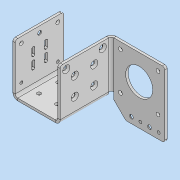
# Autodesk Inventor part: Gantry_Angle
Saved by Autodesk Inventor 2020 (Build 240168000, 168)
## iProperties
Created: 2021-05-02
Part Number: Gantry_Angle
Material: 一般
Document SubType Name: Sheet Metal
Designer: ken113
Density: 1 g/cm^3
Sheet Metal Rule: Default_mm
Appearance: 既定
Author: ken113
Autodesk Inventor part; units mm, degrees
ref_plane "YZ Plane" through (0, 0, 0) normal (1, 0, 0) x (0, 1, 0)
ref_plane "XZ Plane" through (0, 0, 0) normal (0, 1, 0) x (-1, 0, 0)
ref_plane "XY Plane" through (0, 0, 0) normal (0, 0, 1) x (1, 0, 0)
sketch "スケッチ1" plane through (0, 0, 0) normal (0, 1, 0) x (-1, 0, 0)
  line L0 (15, 20) -> (-20, 20)
  line L1 (-20, 20) -> (-20, -20)
  line L2 (-20, -20) -> (15, -20)
  line L3 (15, -20) -> (15, 20)
  point P0 (0, 0)
  dimension "d0" = 15
  dimension "d1" = 40
  dimension "d2" = 20
  dimension "d3" = 20
  measures "d0" distance from line of L3 point (0, 0)
  measures "d1" distance of L0.end L1.end
  measures "d2" distance from line of point (0, 0) L1
  measures "d3" distance from line of point (0, 0) L2
extrude "プレート1" add sketch "スケッチ1" along normal blind 2
sketch "スケッチ2" plane through (0, 2, 0) normal (0, 1, 0) x (1, 0, 0)
  line L0 (7.5, 8) -> (-7.5, 8)
  line L1 (-7.5, 8) -> (-7.5, -8)
  line L2 (-7.5, -8) -> (7.5, -8)
  line L3 (7.5, -8) -> (7.5, 8)
  line L4 (7.5, 8) -> (-7.5, -8) construction
  line L5 (-7.5, 8) -> (7.5, -8) construction
  point P0 (0, 0)
  dimension "d5" = 15
  dimension "d6" = 16
  constraints: 12 end point, 2 midpoint, 2 parallel, 1 horizontal, 1 perpendicular
  measures "d5" distance of L2.end L1.end
  measures "d6" distance of L1.end L0.end
hole "穴1" at (-7.5, 2, 8) at (7.5, 2, 8) at (7.5, 2, -8) at (-7.5, 2, -8) direction (0, -1, 0) diameter 3.2 depth 2 tip angle 118
sketch "スケッチ3" plane through (-15, 2, 20) normal (-1, 0, 0) x (0, -1, 0)
  line L0 (0, -40) -> (0, 0)
  line L1 (0, 0) -> (-40.5, 0)
  line L2 (-40.5, 0) -> (-40.5, -40)
  line L3 (-40.5, -40) -> (0, -40)
  constraints: 6 end point, 1 horizontal, 1 perpendicular, 1 vertical
edge flange "フランジ1" height 42.5 angle 90 thickness 2 bend radius 2 thickness toward (-1, 0, 0) relief straight relief width 2 relief depth 1 corner gap 2 corner form 0 edges at (-15, 2, 0) (20, 2, 0) wall of the first edge with corners at (-15, 2, -20) (-15, 2, 20) (-15, 42.5, 20) (-15, 42.5, -20)
bend "曲げ1"
corner "コーナー1"
sketch "スケッチ5" plane through (22, 42.5, 20) normal (1, 0, 0) x (0, 0, -1)
  line L0 (12, -28) -> (28, -28)
  line L1 (28, -28) -> (28, -13)
  line L2 (28, -13) -> (12, -13)
  line L3 (12, -13) -> (12, -28)
  line L4 (12, -28) -> (28, -13) construction
  line L5 (28, -28) -> (12, -13) construction
  line L6 (0, -38.5) -> (40, -38.5) projected
  point P0 (20, -42.5)
  point P1 (20, -20.5)
  point P2 (20, -20.5)
  dimension "d34" = 16
  dimension "d35" = 15
  dimension "d36" = 10.5
  constraints: 12 end point, 3 midpoint, 2 parallel, 1 horizontal, 1 perpendicular, 1 vertical alignment
  measures "d34" distance of L1.end L2.end
  measures "d35" distance of L0.end L1.end
  measures "d36" distance between parallel lines of L0 L6
hole "穴2" at (22, 29.5, 8) at (22, 29.5, -8) at (22, 14.5, -8) at (22, 14.5, 8) direction (-1, 0, 0) diameter 3.2 depth 2 tip angle 118 countersink diameter 6 countersink angle 90
sketch "スケッチ6" plane through (24, 42.5, -22) normal (0, 0, -1) x (-1, 0, 0)
  line L0 (0, -38.5) -> (0, 0)
  line L1 (0, 0) -> (-42, 0)
  line L2 (-42, 0) -> (-42, -38.5)
  line L3 (-42, -38.5) -> (0, -38.5)
  constraints: 6 end point, 1 horizontal, 1 perpendicular, 1 vertical
edge flange "フランジ3" height 46 angle 90 thickness 2 bend radius 2 thickness toward (0, 0, -1) relief straight relief width 2 relief depth 1 edges at (22, 23.25, -20) wall of the first edge with corners at (24, 4, -22) (24, 42.5, -22) (66, 42.5, -22) (66, 4, -22)
bend "曲げ3"
corner "コーナー3"
sketch "スケッチ7" plane through (66, 4, -24) normal (0, -1, 0) x (1, 0, 0)
  line L0 (-42, 2) -> (-42, 0) projected
  line L1 (-42, 0) -> (0, 0) projected
  line L2 (0, 2) -> (0, 0) projected
  line L3 (0, 2) -> (-42, 2) projected
  point P0 (-66, 24)
extrude "押し出し1" add sketch "スケッチ7" along normal blind 15.5
sketch "スケッチ8" plane through (66, 42.5, -24) normal (0, 0, -1) x (-1, 0, 0)
  circle A0 centre (21, -21) radius 11.15
  line L0 (42, -38.5) -> (42, 0) projected
  line L1 (5.5, -36.5) -> (36.5, -36.5)
  line L2 (36.5, -36.5) -> (36.5, -5.5)
  line L3 (36.5, -5.5) -> (5.5, -5.5)
  line L4 (5.5, -5.5) -> (5.5, -36.5)
  line L5 (5.5, -36.5) -> (36.5, -5.5) construction
  line L6 (36.5, -36.5) -> (5.5, -5.5) construction
  circle A1 centre (5.5, -5.5) radius 1.6
  circle A2 centre (36.5, -5.5) radius 1.6
  circle A3 centre (36.5, -36.5) radius 1.6
  circle A4 centre (5.5, -36.5) radius 1.6
  line L7 (0, 0) -> (42, 0) projected
  point P0 (66, -42.5)
  dimension "d56" = 22.3
  dimension "d57" = 21
  dimension "d58" = 31
  dimension "d59" = 31
  dimension "d60" = 3.2
  dimension "d61" = 3.2
  dimension "d62" = 3.2
  dimension "d63" = 3.2
  dimension "d66" = 21
  constraints: 12 end point, 5 centre point, 4 coincident, 2 midpoint, 2 parallel, 1 horizontal, 1 perpendicular
  measures "d56" diameter of A0
  measures "d57" distance from line of A0.centre L0
  measures "d58" distance of L3.end L2.end
  measures "d59" distance of L2.end L1.end
  measures "d60" diameter of A1
  measures "d61" diameter of A2
  measures "d62" diameter of A3
  measures "d63" diameter of A4
  measures "d66" distance from line of L7 A0.centre
extrude "押し出し2" cut sketch "スケッチ8" against normal blind 25.5 contours A0 | L4 A4 L1 | L1 A4 L4 | A3 L2 L1 | L1 L2 A3 | A1 L3 L4 | L4 L3 A1 | A2 L3 L2 | L2 L3 A2
sketch "スケッチ9" plane through (66, 42.5, -24) normal (0, 0, -1) x (-1, 0, 0)
  circle A0 centre (5.5, -36.5) radius 1.6 projected
  circle A1 centre (36.5, -36.5) radius 1.6 projected
  circle A2 centre (5.5, -5.5) radius 1.6 projected
  circle A3 centre (36.5, -5.5) radius 1.6 projected
  circle A4 centre (21, -21) radius 11.15 projected
  line L0 (42, -38.5) -> (42, 0) projected
  line L1 (0, 0) -> (42, 0) projected
  line L2 (0, 0) -> (0, -54) projected
  line L3 (42, -54) -> (0, -54) projected
  line L4 (42, -38.5) -> (42, -54) projected
  point P0 (66, -42.5)
  point P1 (5, -49)
  point P2 (20, -49)
  dimension "d67" = 5
  dimension "d69" = 5
  dimension "d77" = 15
  constraints: 1 horizontal alignment
  measures "d67" distance from line of point (20, -49) L3
  measures "d69" distance from line of point (5, -49) L2
  measures "d77" distance of point (20, -49) point (5, -49)
hole "穴3" at (61, -6.5, -24) at (46, -6.5, -24) direction (0, 0, 1) diameter 2.459 end through all thread size "M3x0.5" class "6H" standard "ISO Metric profile"
chamfer "面取り1" distance 10 angle 45 1 edges at (24, -11.5, -23)
sketch "スケッチ10" plane through (22, 4, 20) normal (1, 0, 0) x (0, 0, -1)
  circle A0 centre (28, 10.5) radius 3 projected
  circle A1 centre (12, 25.5) radius 3 projected
  circle A2 centre (28, 25.5) radius 3 projected
  circle A3 centre (12, 10.5) radius 3 projected
  line L0 (0, 0) -> (40, 0) projected
  line L1 (40, 38.5) -> (40, 0) projected
  line L2 (0, 38.5) -> (40, 38.5) projected
  line L3 (0, 0) -> (0, 38.5) projected
  point P0 (20, -4)
  point P1 (5, 33.5)
  point P2 (35, 33.5)
  dimension "d81" = 5
  dimension "d82" = 30
  dimension "d83" = 5
  constraints: 1 horizontal alignment
  measures "d81" distance from line of L2 point (5, 33.5)
  measures "d82" distance of point (35, 33.5) point (5, 33.5)
  measures "d83" distance from line of point (5, 33.5) L3
hole "穴4" at (22, 37.5, 15) at (22, 37.5, -15) direction (-1, 0, 0) diameter 3.2 end through all countersink diameter 6 countersink angle 90
fillet "フィレット1" radius 2 7 edges at (-16, 42.5, -20) (-16, 42.5, 20) (21, 42.5, 20) (66, 42.5, -23) (66, -11.5, -23) (34, -11.5, -23) (24, -1.5, -23)
sketch "スケッチ13" plane through (-17, 4, -20) normal (-1, 0, 0) x (0, 0, 1)
  line L0 (13.5, 26) -> (16, 26)
  line L1 (16, 26) -> (16, 19.5)
  line L2 (16, 19.5) -> (13.5, 19.5)
  line L3 (13.5, 19.5) -> (13.5, 26)
  line L4 (13.5, 16.5) -> (16, 16.5)
  line L5 (16, 16.5) -> (16, 10)
  line L6 (16, 10) -> (13.5, 10)
  line L7 (13.5, 10) -> (13.5, 16.5)
  line L8 (24, 19.5) -> (26.5, 19.5)
  line L9 (26.5, 19.5) -> (26.5, 26)
  line L10 (26.5, 26) -> (24, 26)
  line L11 (24, 26) -> (24, 19.5)
  line L12 (24, 16.5) -> (26.5, 16.5)
  line L13 (26.5, 16.5) -> (26.5, 10)
  line L14 (26.5, 10) -> (24, 10)
  line L15 (24, 10) -> (24, 16.5)
  line L16 (40, -4) -> (0, -4) projected
  line L17 (2, 38.5) -> (38, 38.5) projected
  line L18 (13.5, 26) -> (26.5, 26)
  line L19 (26.5, 26) -> (26.5, 26.25)
  line L20 (26.5, 26.25) -> (13.5, 26.25)
  line L21 (13.5, 26.25) -> (13.5, 26)
  line L22 (13.5, 16.5) -> (26.5, 16.5)
  line L23 (26.5, 16.5) -> (26.5, 16.75)
  line L24 (26.5, 16.75) -> (13.5, 16.75)
  line L25 (13.5, 16.75) -> (13.5, 16.5)
  line L26 (13.5, 19.5) -> (26.5, 19.5)
  line L27 (26.5, 19.5) -> (26.5, 19.25)
  line L28 (26.5, 19.25) -> (13.5, 19.25)
  line L29 (13.5, 19.25) -> (13.5, 19.5)
  line L30 (13.5, 10) -> (26.5, 10)
  line L31 (26.5, 10) -> (26.5, 9.75)
  line L32 (26.5, 9.75) -> (13.5, 9.75)
  line L33 (13.5, 9.75) -> (13.5, 10)
  line L34 (16, 26.25) -> (24, 26.25)
  line L35 (24, 26.25) -> (24, 9.75)
  line L36 (24, 9.75) -> (16, 9.75)
  line L37 (16, 9.75) -> (16, 26.25)
  point P0 (20, -4)
  point P1 (26.5, 26.125)
  point P2 (24, 16.75)
  point P3 (24, 19.25)
  point P4 (16, 19.25)
  point P5 (16, 9.75)
  point P6 (16, 10)
  point P7 (16, 16.5)
  point P8 (16, 16.75)
  dimension "d110" = 6.5
  dimension "d111" = 6.5
  dimension "d112" = 2.5
  dimension "d113" = 2.5
  dimension "d114" = 14
  dimension "d115" = 12.5
  dimension "d116" = 8
  dimension "d117" = 4
  dimension "d118" = 7
  dimension "d119" = 0.25
  dimension "d120" = 7
  dimension "d121" = 0.25
  constraints: 72 end point, 18 parallel, 9 horizontal, 9 perpendicular, 9 vertical alignment, 7 point on line, 4 horizontal alignment, 1 coincident, 1 midpoint
  measures "d110" distance of L8.end L9.end
  measures "d111" distance of L12.end L13.end
  measures "d112" distance of L5.end L6.end
  measures "d113" distance of L13.end L14.end
  measures "d114" distance between parallel lines of L6 L16
  measures "d115" distance between parallel lines of L0 L17
  measures "d116" distance between parallel lines of L15 L5
  measures "d117" distance from line of point (20, -4) L5
  measures "d118" distance between parallel lines of L28 L20
  measures "d119" distance between parallel lines of L26 L28
  measures "d120" distance between parallel lines of L24 L32
  measures "d121" distance between parallel lines of L30 L32
extrude "押し出し3" cut sketch "スケッチ13" against normal blind 10 contours L21 L20 L37 L0 | L0 L1 L2 L3 | L2 L37 L28 L29 | L35 L20 L19 L10 | L10 L9 L8 L11 | L8 L27 L28 L35 | L37 L4 L25 L24 | L24 L23 L12 L35 | L5 L6 L7 L4 | L12 L13 L14 L15 | L37 L32 L33 L6 | L14 L31 L32 L35
fillet "フィレット2" radius 1 16 edges at (-16, 23.25, -6.5) (-16, 30.25, -6.5) (-16, 30.25, 4) (-16, 30.25, 6.5) (-16, 23.25, 6.5) (-16, 23.25, 4) (-16, 20.75, 4) (-16, 20.75, 6.5) (-16, 13.75, 6.5) (-16, 13.75, 4) (-16, 13.75, -6.5) (-16, 20.75, -6.5) (-16, 13.75, -4) (-16, 20.75, -4) (-16, 23.25, -4) (-16, 30.25, -4)
sketch "スケッチ14" plane through (-17, 4, -20) normal (-1, 0, 0) x (0, 0, 1)
  line L0 (25, 26.25) -> (25.5, 26.25) projected
  arc A0 (26.5, 25.25) -> (25.5, 26.25) centre (25.5, 25.25) ccw projected
  line L1 (26.5, 25.25) -> (26.5, 20.25) projected
  arc A1 (25.5, 19.25) -> (26.5, 20.25) centre (25.5, 20.25) ccw projected
  line L2 (25.5, 19.25) -> (25, 19.25) projected
  arc A2 (24, 20.25) -> (25, 19.25) centre (25, 20.25) ccw projected
  line L3 (24, 20.25) -> (24, 25.25) projected
  arc A3 (25, 26.25) -> (24, 25.25) centre (25, 25.25) ccw projected
  line L4 (14.5, 26.25) -> (15, 26.25) projected
  arc A4 (16, 25.25) -> (15, 26.25) centre (15, 25.25) ccw projected
  line L5 (16, 25.25) -> (16, 20.25) projected
  arc A5 (15, 19.25) -> (16, 20.25) centre (15, 20.25) ccw projected
  line L6 (15, 19.25) -> (14.5, 19.25) projected
  arc A6 (13.5, 20.25) -> (14.5, 19.25) centre (14.5, 20.25) ccw projected
  line L7 (13.5, 20.25) -> (13.5, 25.25) projected
  arc A7 (14.5, 26.25) -> (13.5, 25.25) centre (14.5, 25.25) ccw projected
  line L8 (25, 16.75) -> (25.5, 16.75) projected
  arc A8 (26.5, 15.75) -> (25.5, 16.75) centre (25.5, 15.75) ccw projected
  line L9 (26.5, 15.75) -> (26.5, 10.75) projected
  arc A9 (25.5, 9.75) -> (26.5, 10.75) centre (25.5, 10.75) ccw projected
  line L10 (25.5, 9.75) -> (25, 9.75) projected
  arc A10 (24, 10.75) -> (25, 9.75) centre (25, 10.75) ccw projected
  line L11 (24, 10.75) -> (24, 15.75) projected
  arc A11 (25, 16.75) -> (24, 15.75) centre (25, 15.75) ccw projected
  line L12 (15, 9.75) -> (14.5, 9.75) projected
  arc A12 (13.5, 10.75) -> (14.5, 9.75) centre (14.5, 10.75) ccw projected
  line L13 (13.5, 10.75) -> (13.5, 15.75) projected
  arc A13 (14.5, 16.75) -> (13.5, 15.75) centre (14.5, 15.75) ccw projected
  line L14 (14.5, 16.75) -> (15, 16.75) projected
  arc A14 (16, 15.75) -> (15, 16.75) centre (15, 15.75) ccw projected
  line L15 (16, 15.75) -> (16, 10.75) projected
  arc A15 (15, 9.75) -> (16, 10.75) centre (15, 10.75) ccw projected
  arc A16 (40, 36.5) -> (38, 38.5) centre (38, 36.5) ccw projected
  line L16 (2, 38.5) -> (38, 38.5) projected
  arc A17 (2, 38.5) -> (0, 36.5) centre (2, 36.5) ccw projected
  line L17 (0, 0) -> (0, 36.5) projected
  line L18 (0, 0) -> (40, 0) projected
  line L19 (40, 36.5) -> (40, 0) projected
  line L20 (5, 5.5) -> (35, 5.5)
  line L21 (35, 5.5) -> (35, 33.5)
  line L22 (35, 33.5) -> (5, 33.5)
  line L23 (5, 33.5) -> (5, 5.5)
  line L24 (5, 5.5) -> (35, 33.5) construction
  line L25 (35, 5.5) -> (5, 33.5) construction
  point P0 (20, -4)
  point P1 (20, 19.5)
  point P2 (20, 19.5)
  point P3 (20, 33.5)
  dimension "d125" = 28
  constraints: 12 end point, 4 midpoint, 2 coincident, 2 parallel, 1 horizontal, 1 perpendicular, 1 vertical alignment
  measures "d125" distance of L20.end L21.end
hole "穴7" at (-17, 37.5, 0) at (-17, 9.5, -15) at (-17, 9.5, 15) direction (1, 0, 0) diameter 2.459 depth 8.8 tip angle 118 thread size "M3x0.5" class "6H" standard "ISO Metric profile"
sketch "スケッチ15" plane through (-17, 4, -20) normal (-1, 0, 0) x (0, 0, 1)
  circle A0 centre (20, 33.5) radius 1.2295 projected
  point P0 (20, -4)
hole "穴8" at (-17, 37.5, 0) direction (1, 0, 0) diameter 3.2 depth 2 tip angle 118 countersink diameter 6 countersink angle 90
sketch "スケッチ16" plane through (24, 4, -24) normal (0, 0, -1) x (-1, 0, 0)
  arc A0 (-0.5858, -6.0858) -> (0, -4.6716) centre (-2, -4.6716) ccw projected
  line L0 (0, 0) -> (0, -4.6716) projected
  line L1 (0, 0) -> (0, 38.5) projected
  line L2 (-40, 38.5) -> (0, 38.5) projected
  arc A1 (-40, 38.5) -> (-42, 36.5) centre (-40, 36.5) ccw projected
  line L3 (-42, 36.5) -> (-42, -13.5) projected
  arc A2 (-42, -13.5) -> (-40, -15.5) centre (-40, -13.5) ccw projected
  line L4 (-10.8284, -15.5) -> (-40, -15.5) projected
  arc A3 (-10.8284, -15.5) -> (-9.4142, -14.9142) centre (-10.8284, -13.5) ccw projected
  line L5 (-0.5858, -6.0858) -> (-9.4142, -14.9142) projected
  circle A4 centre (-37, -10.5) radius 1.2295 projected
  circle A5 centre (-22, -10.5) radius 1.2295 projected
  circle A6 centre (-36.5, 2) radius 1.6 projected
  circle A7 centre (-5.5, 2) radius 1.6 projected
  circle A8 centre (-36.5, 33) radius 1.6 projected
  circle A9 centre (-5.5, 33) radius 1.6 projected
  circle A10 centre (-21, 17.5) radius 11.15 projected
  point P0 (24, -4)
  point P1 (-29.5, -10.5)
  point P2 (-14.5, -10.5)
  dimension "d140" = 7.5
  dimension "d141" = 15
  constraints: 2 horizontal alignment
  measures "d140" distance of A5.centre point (-29.5, -10.5)
  measures "d141" distance of point (-14.5, -10.5) point (-29.5, -10.5)
hole "穴9" at (53.5, -6.5, -24) at (38.5, -6.5, -24) direction (0, 0, 1) diameter 3.2 depth 2 tip angle 118 countersink diameter 6 countersink angle 90
equation "\"d12\" = Thickness"
equation "\"d42\" = Thickness"
equation "\"d117\" = 0.5 * d116"
equation "\"d138\" = Thickness"
equation "\"d147\" = Thickness"
equation "\"d4\" = Thickness"
equation "\"d14\" = BendReliefWidth"
equation "\"d15\" = BendReliefDepth"
equation "\"d16\" = MinimumRemnant"
equation "\"d17\" = TransitionRadius"
equation "\"d20\" = BendRadius"
equation "\"d21\" = CornerReliefSize"
equation "\"d22\" = GapSize"
equation "\"d23\" = JacobiRadiusSize"
equation "\"d44\" = BendReliefWidth"
equation "\"d45\" = BendReliefDepth"
equation "\"d46\" = MinimumRemnant"
equation "\"d47\" = TransitionRadius"
equation "\"d50\" = BendRadius"
equation "\"d51\" = CornerReliefSize"
equation "\"d52\" = GapSize"
equation "\"d53\" = JacobiRadiusSize"
equation "\"d3\" = 0.5 * d1"
equation "\"BendRadius\" = Thickness"
equation "\"BendReliefWidth\" = Thickness"
equation "\"BendReliefDepth\" = 0.5 * Thickness"
equation "\"CornerReliefSize\" = 4 * Thickness"
equation "\"MinimumRemnant\" = 2 * Thickness"
equation "\"TransitionRadius\" = BendRadius"
equation "\"JacobiRadiusSize\" = BendRadius"
equation "\"GapSize\" = Thickness"
equation "\"Thickness\" = 2"
